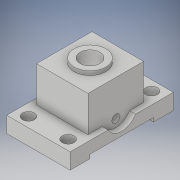
# Autodesk Inventor part: 模型3
Saved by Autodesk Inventor 2018 (Build 220112000, 112)
## iProperties
Created: 2020-05-06
Part Number: 模型3
Material: 常规
Document SubType Name: Modeling
Designer: PC
Density: 1 g/cm^3
Appearance: 默认
Author: PC
Autodesk Inventor part; units mm, degrees
ref_plane "YZ Plane" through (0, 0, 0) normal (1, 0, 0) x (0, 1, 0)
ref_plane "XZ Plane" through (0, 0, 0) normal (0, 1, 0) x (-1, 0, 0)
ref_plane "XY Plane" through (0, 0, 0) normal (0, 0, 1) x (1, 0, 0)
sketch "草图1" plane through (0, 0, 0) normal (0, 1, 0) x (-1, 0, 0)
  line L0 (-16, 26) -> (16, 26)
  line L1 (16, 26) -> (16, -26)
  line L2 (16, -26) -> (-16, -26)
  line L3 (-16, -26) -> (-16, 26)
  line L4 (-16, 26) -> (16, -26) construction
  line L5 (16, 26) -> (-16, -26) construction
  point P0 (0, 0)
  dimension "d0" = 52
  dimension "d1" = 32
  constraints: 12 end point, 2 midpoint, 2 parallel, 1 horizontal, 1 perpendicular
  measures "d0" distance of L0.end L1.end
  measures "d1" distance of L1.end L2.end
extrude "拉伸1" add sketch "草图1" along normal blind 8
sketch "草图2" plane through (0, 8, 0) normal (0, 1, 0) x (1, 0, 0)
  line L0 (13, -14) -> (-13, -14)
  line L1 (-13, -14) -> (-13, 14)
  line L2 (-13, 14) -> (13, 14)
  line L3 (13, 14) -> (13, -14)
  line L4 (13, -14) -> (-13, 14) construction
  line L5 (-13, -14) -> (13, 14) construction
  point P0 (0, 0)
  dimension "d4" = 28
  dimension "d5" = 26
  constraints: 12 end point, 2 midpoint, 2 parallel, 1 horizontal, 1 perpendicular
  measures "d4" distance of L0.end L1.end
  measures "d5" distance of L1.end L2.end
extrude "拉伸2" add sketch "草图2" along normal blind 18
sketch "草图3" plane through (16, 0, 26) normal (1, 0, 0) x (0, 0, -1)
  line L0 (10, -2) -> (42, -2)
  line L1 (42, -2) -> (42, 2)
  line L2 (42, 2) -> (10, 2)
  line L3 (10, 2) -> (10, -2)
  line L4 (10, -2) -> (42, 2) construction
  line L5 (42, -2) -> (10, 2) construction
  line L6 (52, 0) -> (0, 0) projected
  point P0 (26, 0)
  dimension "d8" = 2
  dimension "d9" = 32
  constraints: 12 end point, 2 midpoint, 2 parallel, 1 horizontal, 1 perpendicular
  measures "d8" distance between parallel lines of L6 L2
  measures "d9" distance of L0.start L0.end
extrude "拉伸3" cut sketch "草图3" against normal through all
sketch "草图4" plane through (16, 0, -26) normal (1, 0, 0) x (0, 0, -1)
  line L0 (-40, 26) -> (-12, 26) construction
  line L1 (-26, 26) -> (-26, 12) construction
  circle A0 centre (-26, 12) radius 8
  point P0 (-26, 0)
  dimension "d12" = 14
  dimension "d13" = 16
  constraints: 2 end point, 1 centre point, 1 coincident, 1 midpoint, 1 vertical
  measures "d12" distance of L1.start L1.end
  measures "d13" diameter of A0
extrude "拉伸4" cut sketch "草图4" against normal up to surface (3 mm away)
sketch "草图5" plane through (0, 8, 0) normal (0, 1, 0) x (1, 0, 0)
  line L0 (10, -21) -> (-10, -21) construction
  line L1 (-10, -21) -> (-10, 21) construction
  line L2 (-10, 21) -> (10, 21) construction
  line L3 (10, 21) -> (10, -21) construction
  line L4 (10, -21) -> (-10, 21) construction
  line L5 (-10, -21) -> (10, 21) construction
  circle A0 centre (-10, -21) radius 3
  circle A1 centre (-10, 21) radius 3
  circle A2 centre (10, 21) radius 3
  circle A3 centre (10, -21) radius 3
  line L6 (16, -26) -> (-16, -26) projected
  point P0 (0, 0)
  dimension "d16" = 6
  dimension "d18" = 20
  dimension "d19" = 5
  constraints: 12 end point, 4 centre point, 4 coincident, 3 equal radius, 2 midpoint, 2 parallel, 1 horizontal, 1 perpendicular
  measures "d16" diameter of A0
  measures "d18" distance of L1.end L2.end
  measures "d19" distance from line of L6 A3.centre
extrude "拉伸5" cut sketch "草图5" against normal blind 18
sketch "草图6" plane through (0, 0, 0) normal (0, -1, 0) x (1, 0, 0)
  line L0 (-10, 10) -> (10, 10)
  line L1 (10, 10) -> (10, -10)
  line L2 (10, -10) -> (-10, -10)
  line L3 (-10, -10) -> (-10, 10)
  line L4 (-10, 10) -> (10, -10) construction
  line L5 (10, 10) -> (-10, -10) construction
  point P0 (0, 0)
  dimension "d22" = 20
  dimension "d23" = 20
  constraints: 12 end point, 2 midpoint, 2 parallel, 1 horizontal, 1 perpendicular
  measures "d22" distance of L0.end L1.end
  measures "d23" distance of L1.end L2.end
extrude "拉伸6" cut sketch "草图6" against normal blind 24
sketch "草图7" plane through (13, 8, -14) normal (1, 0, 0) x (0, 0, -1)
  line L0 (0, 18) -> (-28, 18) construction
  line L1 (-14, 18) -> (-14, 0) construction
  circle A0 centre (-14, 0) radius 2
  point P0 (-14, -8)
  dimension "d26" = 18
  dimension "d27" = 4
  constraints: 2 end point, 1 centre point, 1 coincident, 1 midpoint, 1 vertical
  measures "d26" distance of L1.start L1.end
  measures "d27" diameter of A0
extrude "拉伸7" cut sketch "草图7" against normal up to surface (3 mm away)
sketch "草图8" plane through (0, 26, 0) normal (0, 1, 0) x (1, 0, 0)
  circle A0 centre (0, 0) radius 8
  dimension "d30" = 16
  constraints: 1 centre point, 1 coincident
  measures "d30" diameter of A0
extrude "拉伸8" add sketch "草图8" along normal blind 2 and the other way blind 12
sketch "草图9" plane through (0, 28, 0) normal (0, 1, 0) x (1, 0, 0)
  circle A0 centre (0, 0) radius 5
  dimension "d35" = 10
  constraints: 1 centre point, 1 coincident
  measures "d35" diameter of A0
extrude "拉伸9" cut sketch "草图9" against normal blind 12
sketch "草图10" plane through (0, 16, 0) normal (0, 1, 0) x (1, 0, 0)
  circle A0 centre (0, 0) radius 3
  dimension "d38" = 6
  constraints: 1 centre point, 1 coincident
  measures "d38" diameter of A0
extrude "拉伸10" cut sketch "草图10" against normal blind 12
